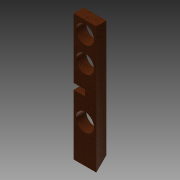
# Autodesk Inventor part: stand1
Saved by Autodesk Inventor 2015 (Build 190159000, 159)
## iProperties
Created: 2014-07-19
Part Number: stand1
Material: Wood (Walnut)
Document SubType Name: Modeling
Designer: pc
Density: 0.55 g/cm^3
Appearance: Walnut - Natural Polished
Author: pc
Autodesk Inventor part; units mm, degrees
ref_plane "YZ Plane" through (0, 0, 0) normal (1, 0, 0) x (0, 1, 0)
ref_plane "XZ Plane" through (0, 0, 0) normal (0, 1, 0) x (-1, 0, 0)
ref_plane "XY Plane" through (0, 0, 0) normal (0, 0, 1) x (1, 0, 0)
sketch "Sketch1" plane through (0, 0, 0) normal (0, 1, 0) x (-1, 0, 0)
  line L0 (22.5, 125) -> (-22.5, 125)
  line L1 (-22.5, 125) -> (-22.5, -125)
  line L2 (-22.5, -125) -> (22.5, -125)
  line L3 (22.5, -125) -> (22.5, 125)
  line L4 (22.5, 125) -> (-22.5, -125) construction
  line L5 (-22.5, 125) -> (22.5, -125) construction
  point P0 (0, 0)
  dimension "d0" = 250
  dimension "d1" = 45
  constraints: 12 end point, 2 midpoint, 2 parallel, 1 horizontal, 1 perpendicular
  measures "d0" distance of L0.end L1.end
  measures "d1" distance of L0.start L0.end
extrude "Extrusion1" add sketch "Sketch1" along normal blind 20
sketch "Sketch2" plane through (0, 0, 0) normal (0, -1, 0) x (1, 0, 0)
  circle A0 centre (0, 100) radius 17.75
  circle A1 centre (0, 50) radius 17.75
  circle A2 centre (0, -50) radius 17.75
  line L0 (0, 50) -> (0, -50) construction
  line L1 (0, 100) -> (0, 50) construction
  line L2 (0, 0) -> (0, 148) construction
  line L3 (-35.7491, 0) -> (26.8031, 0) construction
  line L4 (0, -6) -> (-22.5, -6)
  line L5 (-22.5, -6) -> (-22.5, 6)
  line L6 (-22.5, 6) -> (0, 6)
  line L7 (0, 6) -> (0, -6)
  line L8 (0, -6) -> (-22.5, 6) construction
  line L9 (-22.5, -6) -> (0, 6) construction
  line L10 (-18, 98) -> (-18, -100) projected
  line L11 (-22.5, 125) -> (22.5, 125) projected
  line L12 (-22.5, -125) -> (-22.5, 125) projected
  point P0 (0, 75)
  point P1 (-11.5, 0)
  point P2 (-11.25, 0)
  point P3 (-25, -148)
  point P4 (-16, 100)
  dimension "d9" = 35.5
  dimension "d10" = 35.5
  dimension "d11" = 35.5
  dimension "d12" = 50
  dimension "d13" = 100
  dimension "d16" = 12
  dimension "d36" = 25
  constraints: 20 end point, 3 centre point, 3 midpoint, 3 point on line, 2 collinear, 2 horizontal, 2 vertical, 1 coincident, 1 parallel, 1 perpendicular, 2 other
  measures "d9" diameter of A0
  measures "d10" diameter of A1
  measures "d11" diameter of A2
  measures "d12" distance of L0.start L1.start
  measures "d13" distance of A2.centre L0.start
  measures "d16" distance between parallel lines of L4 L6
sketch "Sketch4" plane through (22.5, 0, 125) normal (1, 0, 0) x (0, 0, -1)
  line L0 (250, 0) -> (230, 20)
  line L1 (0, 20) -> (250, 20) projected
  line L2 (250, 0) -> (250, 20)
  point P0 (125, 0)
  dimension "d29" = 45
  constraints: 4 end point, 1 perpendicular, 1 point on line
  measures "d29" angle of L1 L0
extrude "Extrusion4" cut sketch "Sketch4" against normal through all
extrude "Extrusion5" cut sketch "Sketch2" against normal through all
equation "\"d9\" = d11"
equation "\"d10\" = d11"
equation "\"d13\" = 2 * d12"
body "Solid1"
